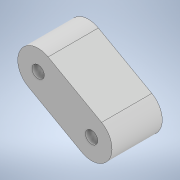
# Autodesk Inventor part: leg_fixer_2
Saved by Autodesk Inventor 2020 (Build 240168000, 168)
## iProperties
Created: 2020-08-19
Part Number: leg_fixer_2
Material: Generic
Document SubType Name: Modeling
Designer: psrobotics
Density: 1 g/cm^3
Appearance: Default
Author: psrobotics
Autodesk Inventor part; units mm, degrees
ref_plane "YZ Plane" through (0, 0, 0) normal (1, 0, 0) x (0, 1, 0)
ref_plane "XZ Plane" through (0, 0, 0) normal (0, 1, 0) x (-1, 0, 0)
sketch "Sketch1" plane through (0, 0, 0) normal (0, 0, 1) x (1, 0, 0)
  line L0 (86.516, -0.3214) -> (114.7595, -23.8164) projected
  arc A0 (113.4805, -27.354) -> (114.7595, -23.8164) centre (113.4805, -25.354) ccw projected
  line L1 (113.4805, -27.354) -> (84.3159, -27.354) projected
  arc A1 (80.4978, -22.1613) -> (84.3159, -27.354) centre (84.3159, -23.354) ccw projected
  arc A2 (80.4978, -22.1613) -> (83.238, -1.9261) centre (22.2724, -3.9734) ccw projected
  arc A3 (86.516, -0.3214) -> (83.238, -1.9261) centre (85.2369, -1.8589) ccw projected
  arc A4 (123.464, -37.945) -> (119.4703, -38.0751) centre (121.4642, -37.9192) ccw projected
  arc A5 (144.0129, -57.1973) -> (123.464, -37.945) centre (122.1805, -59.9075) ccw projected
  arc A6 (144.143, -61.191) -> (144.0129, -57.1973) centre (144.1688, -59.1912) ccw projected
  arc A7 (124.8907, -81.7399) -> (144.143, -61.191) centre (122.1805, -59.9075) ccw projected
  arc A8 (120.8969, -81.87) -> (124.8907, -81.7399) centre (122.8968, -81.8958) ccw projected
  arc A9 (100.3481, -62.6177) -> (120.8969, -81.87) centre (122.1805, -59.9075) ccw projected
  arc A10 (100.218, -58.6239) -> (100.3481, -62.6177) centre (100.1921, -60.6238) ccw projected
  arc A11 (119.4703, -38.0751) -> (100.218, -58.6239) centre (122.1805, -59.9075) ccw projected
  arc A12 (87.2274, -61.7195) -> (88.373, -68.9659) centre (122.1805, -59.9075) ccw projected
  arc A13 (85.8324, -71.3887) -> (88.373, -68.9659) centre (86.4412, -69.4836) ccw projected
  line L2 (85.8324, -71.3887) -> (52.5887, -60.766) projected
  arc A14 (52.2157, -57.1184) -> (52.5887, -60.766) centre (53.1975, -58.8609) ccw projected
  arc A15 (52.2157, -57.1184) -> (67.1926, -45.2429) centre (22.2724, -3.9734) ccw projected
  arc A16 (72.896, -45.0519) -> (67.1926, -45.2429) centre (70.1382, -47.9491) ccw projected
  line L3 (72.896, -45.0519) -> (84.7539, -56.3391) projected
  arc A17 (87.2274, -61.7195) -> (84.7539, -56.3391) centre (79.2381, -62.1337) ccw projected
  circle A18 centre (-5.6495, 11.6589) radius 2.05 projected
  circle A19 centre (-18.7379, 18.9865) radius 2.05 projected
  line L4 (2.166, 24.8708) -> (-5.7638, 34.6785) projected
  arc A20 (-5.0374, 39.0984) -> (-5.7638, 34.6785) centre (-3.431, 36.5647) ccw projected
  arc A21 (4.796, 43.9388) -> (-5.0374, 39.0984) centre (22.2724, -3.9734) ccw projected
  arc A22 (8.7012, 41.9703) -> (4.796, 43.9388) centre (5.8241, 41.1205) ccw projected
  line L5 (8.7012, 41.9703) -> (12.2517, 29.9506) projected
  arc A23 (10.4645, 26.3057) -> (12.2517, 29.9506) centre (9.3746, 29.1007) ccw projected
  arc A24 (10.4645, 26.3057) -> (6.0009, 24.16) centre (22.2724, -3.9734) ccw projected
  arc A25 (2.166, 24.8708) -> (6.0009, 24.16) centre (4.4989, 26.757) ccw projected
  line L6 (21.3733, 31.3882) -> (21.0547, 43.9173) projected
  arc A26 (24.1651, 46.9915) -> (21.0547, 43.9173) centre (24.0537, 43.9936) ccw projected
  arc A27 (35.0106, 45.4102) -> (24.1651, 46.9915) centre (22.2724, -3.9734) ccw projected
  arc A28 (37.0613, 41.4281) -> (35.0106, 45.4102) centre (34.2613, 42.5053) ccw projected
  line L7 (37.0613, 41.4281) -> (32.5324, 29.6567) projected
  arc A29 (29.1021, 27.8009) -> (32.5324, 29.6567) centre (29.7325, 30.7339) ccw projected
  arc A30 (29.1021, 27.8009) -> (24.1948, 28.4697) centre (22.2724, -3.9734) ccw projected
  arc A31 (21.3733, 31.3882) -> (24.1948, 28.4697) centre (24.3723, 31.4645) ccw projected
  line L8 (37.199, 27.8613) -> (41.7278, 39.6327) projected
  arc A32 (45.9187, 41.2135) -> (41.7278, 39.6327) centre (44.5277, 38.5555) ccw projected
  arc A33 (55.0274, 35.1177) -> (45.9187, 41.2135) centre (22.2724, -3.9734) ccw projected
  arc A34 (55.2752, 30.7515) -> (55.0274, 35.1177) centre (53.1006, 32.8182) ccw projected
  line L9 (55.2752, 30.7515) -> (46.641, 21.6668) projected
  arc A35 (42.5909, 21.3921) -> (46.641, 21.6668) centre (44.4665, 23.7336) ccw projected
  arc A36 (42.5909, 21.3921) -> (38.5009, 24.1849) centre (22.2724, -3.9734) ccw projected
  arc A37 (37.199, 27.8613) -> (38.5009, 24.1849) centre (39.9989, 26.7841) ccw projected
  line L10 (52.4469, 14.4861) -> (59.2911, 18.6731) projected
  arc A38 (63.5177, 17.4994) -> (59.2911, 18.6731) centre (60.8567, 16.114) ccw projected
  arc A39 (66.9215, 9.0155) -> (63.5177, 17.4994) centre (22.2724, -3.9734) ccw projected
  arc A40 (64.5079, 5.2141) -> (66.9215, 9.0155) centre (64.0409, 8.1775) ccw projected
  line L11 (64.5079, 5.2141) -> (56.5269, 3.9563) projected
  arc A41 (53.2046, 5.9991) -> (56.5269, 3.9563) centre (56.0599, 6.9197) ccw projected
  arc A42 (53.2046, 5.9991) -> (51.3302, 10.5833) centre (22.2724, -3.9734) ccw projected
  arc A43 (52.4469, 14.4861) -> (51.3302, 10.5833) centre (54.0124, 11.927) ccw projected
  line L12 (57.3053, -0.9828) -> (65.2864, 0.2751) projected
  arc A44 (68.7521, -2.5997) -> (65.2864, 0.2751) centre (65.7534, -2.6883) ccw projected
  arc A45 (68.1227, -11.7192) -> (68.7521, -2.5997) centre (22.2724, -3.9734) ccw projected
  arc A46 (64.4621, -14.1361) -> (68.1227, -11.7192) centre (65.1646, -11.2195) ccw projected
  line L13 (64.4621, -14.1361) -> (56.6618, -12.2571) projected
  arc A47 (54.3988, -8.887) -> (56.6618, -12.2571) centre (57.3643, -9.3405) ccw projected
  arc A48 (54.3988, -8.887) -> (54.7724, -3.9485) centre (22.2724, -3.9734) ccw projected
  arc A49 (57.3053, -0.9828) -> (54.7724, -3.9485) centre (57.7724, -3.9462) ccw projected
  line L14 (53.346, -20.8755) -> (64.3558, -26.8641) projected
  arc A50 (65.463, -31.0949) -> (64.3558, -26.8641) centre (62.9223, -29.4995) ccw projected
  arc A51 (58.6707, -39.6968) -> (65.463, -31.0949) centre (22.2724, -3.9734) ccw projected
  arc A52 (54.1968, -39.4816) -> (58.6707, -39.6968) centre (56.5296, -37.5954) ccw projected
  line L15 (54.1968, -39.4816) -> (46.2669, -29.6738) projected
  arc A53 (46.3749, -25.7752) -> (46.2669, -29.6738) centre (48.5998, -27.7876) ccw projected
  arc A54 (46.3749, -25.7752) -> (49.4077, -21.8598) centre (22.2724, -3.9734) ccw projected
  arc A55 (53.346, -20.8755) -> (49.4077, -21.8598) centre (51.9125, -23.5108) ccw projected
  line L16 (42.3788, -32.8175) -> (50.3087, -42.6252) projected
  arc A56 (49.5823, -47.0451) -> (50.3087, -42.6252) centre (47.9758, -44.5114) ccw projected
  arc A57 (39.7488, -51.8855) -> (49.5823, -47.0451) centre (22.2724, -3.9734) ccw projected
  arc A58 (35.8437, -49.917) -> (39.7488, -51.8855) centre (38.7208, -49.0672) ccw projected
  line L17 (35.8437, -49.917) -> (32.2932, -37.8973) projected
  arc A59 (34.0803, -34.2525) -> (32.2932, -37.8973) centre (35.1703, -37.0474) ccw projected
  arc A60 (34.0803, -34.2525) -> (38.5439, -32.1067) centre (22.2724, -3.9734) ccw projected
  arc A61 (42.3788, -32.8175) -> (38.5439, -32.1067) centre (40.0459, -34.7037) ccw projected
  line L18 (23.1715, -39.3349) -> (23.3755, -47.3558) projected
  arc A62 (20.2457, -50.4292) -> (23.3755, -47.3558) centre (20.3765, -47.432) ccw projected
  arc A63 (11.1966, -49.135) -> (20.2457, -50.4292) centre (22.2724, -3.9734) ccw projected
  arc A64 (9.1112, -45.1441) -> (11.1966, -49.135) centre (11.9112, -46.2214) ccw projected
  line L19 (9.1112, -45.1441) -> (12.0124, -37.6034) projected
  arc A65 (15.4428, -35.7477) -> (12.0124, -37.6034) centre (14.8123, -38.6807) ccw projected
  arc A66 (15.4428, -35.7477) -> (20.35, -36.4165) centre (22.2724, -3.9734) ccw projected
  arc A67 (23.1715, -39.3349) -> (20.35, -36.4165) centre (20.1725, -39.4112) ccw projected
  line L20 (7.3459, -35.8081) -> (4.4447, -43.3488) projected
  arc A68 (0.2222, -44.9128) -> (4.4447, -43.3488) centre (1.6448, -42.2715) ccw projected
  arc A69 (-7.3609, -39.808) -> (0.2222, -44.9128) centre (22.2724, -3.9734) ccw projected
  arc A70 (-7.6236, -35.4294) -> (-7.3609, -39.808) centre (-5.449, -37.4961) ccw projected
  line L21 (-7.6236, -35.4294) -> (-2.0962, -29.6136) projected
  arc A71 (1.9539, -29.3388) -> (-2.0962, -29.6136) centre (0.0783, -31.6803) ccw projected
  arc A72 (1.9539, -29.3388) -> (6.0439, -32.1316) centre (22.2724, -3.9734) ccw projected
  arc A73 (7.3459, -35.8081) -> (6.0439, -32.1316) centre (4.5459, -34.7308) ccw projected
  line L22 (-7.9021, -22.4328) -> (-18.5933, -28.9733) projected
  arc A74 (-22.8108, -27.8167) -> (-18.5933, -28.9733) centre (-20.1588, -26.4142) ccw projected
  arc A75 (-26.8641, -17.6335) -> (-22.8108, -27.8167) centre (22.2724, -3.9734) ccw projected
  arc A76 (-24.4408, -13.8666) -> (-26.8641, -17.6335) centre (-23.9738, -16.83) ccw projected
  line L23 (-24.4408, -13.8666) -> (-11.9821, -11.903) projected
  arc A77 (-8.6598, -13.9459) -> (-11.9821, -11.903) centre (-11.515, -14.8664) ccw projected
  arc A78 (-8.6598, -13.9459) -> (-6.7854, -18.53) centre (22.2724, -3.9734) ccw projected
  arc A79 (-7.9021, -22.4328) -> (-6.7854, -18.53) centre (-9.4676, -19.8737) ccw projected
  line L24 (-12.7605, -6.9639) -> (-25.2192, -8.9275) projected
  arc A80 (-28.6837, -6.0885) -> (-25.2192, -8.9275) centre (-25.6863, -5.9641) ccw projected
  arc A81 (-27.9589, 4.8477) -> (-28.6837, -6.0885) centre (22.2724, -3.9734) ccw projected
  arc A82 (-24.3016, 7.2454) -> (-27.9589, 4.8477) centre (-25.0042, 4.3289) ccw projected
  line L25 (-24.3016, 7.2454) -> (-12.117, 4.3104) projected
  arc A83 (-9.854, 0.9403) -> (-12.117, 4.3104) centre (-12.8195, 1.3938) ccw projected
  arc A84 (-9.854, 0.9403) -> (-10.2276, -3.9982) centre (22.2724, -3.9734) ccw projected
  arc A85 (-12.7605, -6.9639) -> (-10.2276, -3.9982) centre (-13.2276, -4.0005) ccw projected
  circle A86 centre (85.7696, -48.6911) radius 2.05 projected
  circle A87 centre (93.5857, -34.7301) radius 2.05 projected
  circle A88 centre (76.5892, -34.383) radius 2.05 projected
  circle A89 centre (151.7223, -75.704) radius 1.5 projected
  circle A90 centre (150.6316, -42.2218) radius 1.5 projected
  circle A91 centre (123.2712, -93.3897) radius 1.5 projected
  circle A92 centre (123.1684, -22.4726) radius 2 projected
  circle A93 centre (91.7471, -81.3441) radius 2 projected
  circle A94 centre (110.6431, -14.2192) radius 2 projected
  circle A95 centre (78.0027, -75.3364) radius 2 projected
  arc A96 (-41.3146, 7.2953) -> (-36.3695, 11.8712) centre (-78.5082, 52.4493) ccw projected
  arc A97 (-32.9898, 9.9939) -> (-36.3695, 11.8712) centre (-34.9289, 10.4839) ccw projected
  arc A98 (-32.9898, 9.9939) -> (-34.2864, 3.1052) centre (22.2724, -3.9734) ccw projected
  arc A99 (-37.576, 1.8381) -> (-34.2864, 3.1052) centre (-36.2709, 3.3536) ccw projected
  arc A100 (-37.576, 1.8381) -> (-40.8614, 3.9267) centre (-46.3856, -8.3913) ccw projected
  arc A101 (-41.3146, 7.2953) -> (-40.8614, 3.9267) centre (-40.043, 5.7516) ccw projected
  arc A102 (-33.319, -18.6649) -> (-28.8077, -30.3754) centre (22.2724, -3.9734) ccw projected
  arc A103 (-31.7455, -32.9222) -> (-28.8077, -30.3754) centre (-30.5844, -31.2938) ccw projected
  line L26 (-31.7455, -32.9222) -> (-43.0588, -24.8558) projected
  arc A104 (-42.4768, -21.313) -> (-43.0588, -24.8558) centre (-41.8977, -23.2274) ccw projected
  arc A105 (-42.4768, -21.313) -> (-36.6892, -17.7843) centre (-46.3856, -8.3913) ccw projected
  arc A106 (-33.319, -18.6649) -> (-36.6892, -17.7843) centre (-35.2527, -19.1759) ccw projected
  line L27 (-64.993, -11.6723) -> (-61.5225, -11.0604) projected
  arc A107 (-59.2669, -12.4314) -> (-61.5225, -11.0604) centre (-61.1752, -13.03) ccw projected
  arc A108 (-59.2669, -12.4314) -> (-52.6012, -20.3753) centre (-46.3856, -8.3913) ccw projected
  arc A109 (-51.6426, -22.8348) -> (-52.6012, -20.3753) centre (-53.522, -22.1507) ccw projected
  line L28 (-51.6426, -22.8348) -> (-52.8479, -26.1463) projected
  arc A110 (-55.6053, -27.2592) -> (-52.8479, -26.1463) centre (-54.7273, -25.4622) ccw projected
  arc A111 (-66.5678, -14.1946) -> (-55.6053, -27.2592) centre (-46.3856, -8.3913) ccw projected
  arc A112 (-64.993, -11.6723) -> (-66.5678, -14.1946) centre (-64.6457, -13.6419) ccw projected
  circle A113 centre (-48.56, 6.9152) radius 2.1 projected
  circle A114 centre (-32.9741, 22.501) radius 2.1 projected
  circle A115 centre (-69.0444, -1.2227) radius 2.1 projected
  circle A116 centre (-24.8362, 42.9855) radius 2.1 projected
  circle A117 centre (-46.3856, -8.3913) radius 8 projected
  line L29 (-28.6687, 48.4472) -> (-17.4995, 54.7179) projected
  arc A118 (-69.8258, 3.2089) -> (-28.6687, 48.4472) centre (-78.5082, 52.4493) ccw projected
  line L30 (-69.8258, 3.2089) -> (-78.128, 1.745) projected
  line L31 (-78.128, 1.745) -> (-74.0482, -21.3924) projected
  line L32 (-74.0482, -21.3924) -> (-71.8042, -20.9967) projected
  arc A119 (-69.7278, -21.9611) -> (-71.8042, -20.9967) centre (-71.4569, -22.9663) ccw projected
  arc A120 (-69.7278, -21.9611) -> (-51.1536, -34.967) centre (-46.3856, -8.3913) ccw projected
  arc A121 (-49.5371, -36.5883) -> (-51.1536, -34.967) centre (-51.5067, -36.9355) ccw projected
  line L33 (-49.5371, -36.5883) -> (-49.1414, -38.8323) projected
  line L34 (-49.1414, -38.8323) -> (-41.7759, -37.5336) projected
  arc A122 (-40.7711, -37.6143) -> (-41.7759, -37.5336) centre (-41.4286, -39.5032) ccw projected
  line L35 (-40.7711, -37.6143) -> (2.4006, -52.6404) projected
  arc A123 (3.6226, -55.2133) -> (2.4006, -52.6404) centre (1.7432, -54.5293) ccw projected
  line L36 (3.6226, -55.2133) -> (1.8974, -59.9532) projected
  line L37 (1.8974, -59.9532) -> (17.5702, -63.2237) projected
  line L38 (17.5702, -63.2237) -> (111.5272, -93.2468) projected
  arc A124 (111.5272, -93.2468) -> (114.3001, -94.0088) centre (122.1805, -59.9075) ccw projected
  arc A125 (115.8487, -95.8923) -> (114.3001, -94.0088) centre (113.8498, -95.9574) ccw projected
  line L39 (115.8487, -95.8923) -> (115.9054, -97.6318) projected
  line L40 (115.9054, -97.6318) -> (130.8974, -97.1434) projected
  line L41 (130.8974, -97.1434) -> (130.8408, -95.404) projected
  arc A126 (132.2635, -93.4236) -> (130.8408, -95.404) centre (132.8397, -95.3388) ccw projected
  arc A127 (132.2635, -93.4236) -> (147.7729, -83.7828) centre (122.1805, -59.9075) ccw projected
  arc A128 (150.1784, -83.3834) -> (147.7729, -83.7828) centre (149.2353, -85.1471) ccw projected
  line L42 (150.1784, -83.3834) -> (151.7131, -84.204) projected
  line L43 (151.7131, -84.204) -> (158.7862, -70.9764) projected
  line L44 (158.7862, -70.9764) -> (157.2515, -70.1557) projected
  arc A129 (156.2478, -67.9334) -> (157.2515, -70.1557) centre (158.1945, -68.392) ccw projected
  arc A130 (156.2478, -67.9334) -> (155.6533, -49.6815) centre (122.1805, -59.9075) ccw projected
  arc A131 (156.5102, -47.3985) -> (155.6533, -49.6815) centre (157.566, -49.0971) ccw projected
  line L45 (156.5102, -47.3985) -> (157.9882, -46.4797) projected
  line L46 (157.9882, -46.4797) -> (150.0693, -33.7404) projected
  line L47 (150.0693, -33.7404) -> (148.5912, -34.6592) projected
  arc A132 (146.1648, -34.4172) -> (148.5912, -34.6592) centre (147.5353, -32.9607) ccw projected
  arc A133 (146.1648, -34.4172) -> (144.5637, -33.0004) centre (122.1805, -59.9075) ccw projected
  line L48 (144.5637, -33.0004) -> (73.8637, 25.8129) projected
  line L49 (73.8637, 25.8129) -> (63.9599, 38.3925) projected
  arc A134 (63.9599, 38.3925) -> (60.1088, 41.8646) centre (22.2724, -3.9734) ccw projected
  line L50 (60.1088, 41.8646) -> (59.4908, 41.1159) projected
  arc A135 (56.7287, 40.804) -> (59.4908, 41.1159) centre (57.9484, 42.389) ccw projected
  arc A136 (56.7287, 40.804) -> (49.4201, 45.5771) centre (22.2724, -3.9734) ccw projected
  arc A137 (48.5953, 48.2316) -> (49.4201, 45.5771) centre (50.3811, 47.3311) ccw projected
  line L51 (48.5953, 48.2316) -> (49.1968, 49.4245) projected
  arc A138 (49.1968, 49.4245) -> (43.4677, 51.9463) centre (22.2724, -3.9734) ccw projected
  line L52 (43.4677, 51.9463) -> (31.8766, 55.0521) projected
  arc A139 (31.8766, 55.0521) -> (25.6541, 55.7327) centre (22.2724, -3.9734) ccw projected
  line L53 (25.6541, 55.7327) -> (25.5786, 54.3989) projected
  arc A140 (23.537, 52.5125) -> (25.5786, 54.3989) centre (23.5818, 54.512) ccw projected
  arc A141 (23.537, 52.5125) -> (14.821, 52.0331) centre (22.2724, -3.9734) ccw projected
  arc A142 (12.5849, 53.6843) -> (14.821, 52.0331) centre (14.5573, 54.0157) ccw projected
  line L54 (12.5849, 53.6843) -> (12.4241, 54.6417) projected
  arc A143 (12.4241, 54.6417) -> (7.3529, 53.5603) centre (22.2724, -3.9734) ccw projected
  line L55 (7.3529, 53.5603) -> (-6.5013, 48.0227) projected
  arc A144 (-8.4026, 48.2499) -> (-6.5013, 48.0227) centre (-7.2436, 49.8798) ccw projected
  line L56 (-8.4026, 48.2499) -> (-17.4995, 54.7179) projected
  circle A145 centre (-71.296, -16.8454) radius 1.5 projected
  circle A146 centre (18.8152, -59.8032) radius 1.5 projected
  circle A147 centre (53.4562, -50.8504) radius 1.5 projected
  circle A148 centre (60.8075, 36.5725) radius 1.5 projected
  circle A149 centre (28.5162, 51.9811) radius 1.5 projected
  circle A150 centre (9.173, 50.4079) radius 1.5 projected
  circle A151 centre (44.8423, 47.6065) radius 1.5 projected
  circle A152 centre (67.2628, -37.2117) radius 1.5 projected
  circle A153 centre (38.1378, -57.9935) radius 1.5 projected
  circle A154 centre (-45.81, -34.6909) radius 1.5 projected
  circle A155 centre (22.2724, -3.9734) radius 24.5 projected
  line L57 (-5.6495, 11.6589) -> (-18.7379, 18.9865) construction
  line L58 (-3.6955, 15.1491) -> (-16.7839, 22.4767)
  line L59 (-20.6919, 15.4963) -> (-7.6035, 8.1686)
  arc A156 (-7.6035, 8.1686) -> (-3.6955, 15.1491) centre (-5.6495, 11.6589) ccw
  arc A157 (-16.7839, 22.4767) -> (-20.6919, 15.4963) centre (-18.7379, 18.9865) ccw
  circle A158 centre (-5.6495, 11.6589) radius 1.5
  circle A159 centre (-18.7379, 18.9865) radius 1.5
  point P0 (0, 0)
  point P1 (-12.1937, 15.3227)
  dimension "d0" = 8
  dimension "d1" = 3
  dimension "d2" = 3
  constraints: 8 end point, 4 centre point, 4 point on circle, 4 tangent, 2 coincident, 1 midpoint, 1 parallel
  measures "d0" diameter of A157
  measures "d1" diameter of A158
  measures "d2" diameter of A159
ref_plane "Work Plane1" through (82.5607, -52.1105, 12.3) normal (0, 0, 1) x (0.9725249, 0.2327991, 0)
extrude "Extrusion1" add sketch "Sketch1" along normal up to surface (12.3 mm away) contours A18 | A19 | A156 L59 A157 L58
thicken "Thicken1" operation add thickness 1 both sides no extend neighbours yes toward (-0.4885077, -0.8725596, 0) faces at (-16.3291, 13.0537, 8.2)
body "Solid1"
